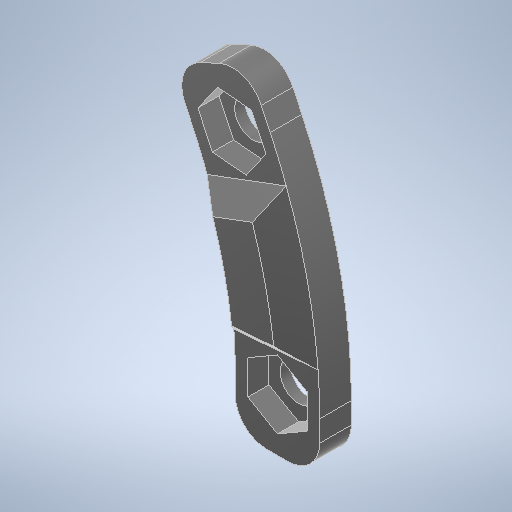
# Autodesk Inventor part: 3D_frame-connect-base2-2
Saved by Autodesk Inventor 2025 (Build 290162000, 162)
## iProperties
Created: 2024-07-30
Part Number: 3D_frame-connect-base2-2
Material: 一般
Document SubType Name: Modeling
Designer: 8326d
Density: 1 g/cm^3
Appearance: 滑らか - 黒
Author: 8326d
Autodesk Inventor part; units mm, degrees
ref_plane "YZ Plane" through (0, 0, 0) normal (1, 0, 0) x (0, 1, 0)
ref_plane "XZ Plane" through (0, 0, 0) normal (0, 1, 0) x (-1, 0, 0)
ref_plane "XY Plane" through (0, 0, 0) normal (0, 0, 1) x (1, 0, 0)
sketch "スケッチ1" plane through (0, 0, 0) normal (0, 0, 1) x (1, 0, 0)
  arc A0 (46, 0) -> (41.6902, 19.4404) centre (0, 0) ccw construction
  line L0 (0, 0) -> (46, 0) construction
  line L1 (0, 0) -> (46, 0) construction
  line L2 (0, 0) -> (41.6902, 19.4404) construction
  arc A1 (50, 0) -> (45.3154, 21.1309) centre (0, 0) ccw
  arc A2 (42, 0) -> (38.0649, 17.75) centre (0, 0) ccw
  line L3 (42, 0) -> (50, 0)
  line L4 (50, 0) -> (50, -5)
  line L5 (50, -5) -> (42, -5)
  line L6 (42, -5) -> (42, 0)
  line L7 (45.3154, 21.1309) -> (38.0649, 17.75)
  line L8 (38.0649, 17.75) -> (35.9518, 22.2815)
  line L9 (35.9518, 22.2815) -> (43.2023, 25.6625)
  line L10 (43.2023, 25.6625) -> (45.3154, 21.1309)
  dimension "d0" = 46
  dimension "d1" = 0
  dimension "d2" = 25
  dimension "d3" = 4
  dimension "d4" = 4
  dimension "d5" = 8
  dimension "d6" = 5
  dimension "d7" = 5
  constraints: 22 end point, 6 point on circle, 4 parallel, 4 point on line, 3 centre point, 3 coincident, 2 horizontal, 2 perpendicular, 1 collinear, 1 horizontal alignment
  measures "d0" radius of A0
  measures "d1" distance between parallel lines of L0 L1
  measures "d2" angle of L0 L2
  measures "d3" radial gap between concentric circles of A2 A0
  measures "d4" radial gap between concentric circles of A0 A1
  measures "d5" distance of L4.end L5.end
  measures "d6" distance of L3.end L4.end
  measures "d7" distance of L7.end L8.end
extrude "押し出し1" add sketch "スケッチ1" along normal blind 3
sketch "スケッチ2" plane through (0, 0, 3) normal (0, 0, 1) x (1, 0, 0)
  arc A0 (46, 0) -> (41.6902, 19.4404) centre (0, 0) ccw construction
  line L0 (0, 0) -> (46, 0) construction
  line L1 (0, 0) -> (46, 0) construction
  line L2 (0, 0) -> (41.6902, 19.4404) construction
  dimension "d10" = 46
  dimension "d11" = 0
  dimension "d12" = 25
  constraints: 6 end point, 3 coincident, 2 point on circle, 1 centre point, 1 collinear, 1 horizontal
  measures "d10" radius of A0
  measures "d11" distance between parallel lines of L0 L1
  measures "d12" angle of L0 L2
hole "穴1" at (41.6902, 19.4404, 3) at (46, 0, 3) direction (0, 0, -1) diameter 3.5 end through all
sketch "スケッチ3" plane through (0, 0, 3) normal (0, 0, 1) x (1, 0, 0)
  circle A0 centre (46, 0) radius 1.75 projected
  line L0 (46, 3.2332) -> (48.8, 1.6166)
  line L1 (48.8, 1.6166) -> (48.8, -1.6166)
  line L2 (48.8, -1.6166) -> (46, -3.2332)
  line L3 (46, -3.2332) -> (43.2, -1.6166)
  line L4 (43.2, -1.6166) -> (43.2, 1.6166)
  line L5 (43.2, 1.6166) -> (46, 3.2332)
  point P0 (0, 0)
  dimension "d20" = 5.6
  constraints: 12 end point, 1 coincident, 1 vertical alignment, 13 other
  measures "d20" distance between parallel lines of L1 L4
extrude "押し出し2" cut sketch "スケッチ3" against normal blind 2
pattern_circular "円形状パターン1" count 2 over 25 about axis through (0, 0, -10) along (0, 0, 1) of "押し出し2"
ref_plane "作業平面1" through (-22.5535, -5, 3) normal (-0.2164396, 0.976296, 0) x (0, 0, -1)
sketch "スケッチ4" plane through (-22.5535, -5, 3) normal (-0.2164396, 0.976296, 0) x (0, 0, -1)
  line L0 (3, -73.1011) -> (0, -73.1011) projected
  line L1 (0, -65.1011) -> (3, -65.1011) projected
  line L2 (0, -65.1011) -> (0, -64.1056) projected
  line L3 (0, -73.1011) -> (0, -65.1011)
  line L4 (0, -65.1011) -> (-2, -67.1011)
  line L5 (-2, -67.1011) -> (-2, -71.1011)
  line L6 (0, -71.9159) -> (0, -73.1011) projected
  line L7 (-2, -71.1011) -> (0, -73.1011)
  line L8 (4, -23.1011) -> (-3, -23.1011) projected
  point P0 (3, -23.1011)
  dimension "d26" = 45
  dimension "d27" = 45
  dimension "d28" = 2
  constraints: 8 end point, 1 parallel, 1 vertical
  measures "d26" angle of L3 L7
  measures "d27" angle of L3 L4
  measures "d28" distance between parallel lines of L3 L5
revolve "回転1" add sketch "スケッチ4" angle 16 mid plane about axis through (0, 0, -10) along (0, 0, 1)
chamfer "面取り1" distance 2 angle 45 2 edges at (43.0869, 16.1095, 5) (45.8582, 3.6091, 5)
fillet "フィレット1" radius 3 4 edges at (43.2023, 25.6625, 1.5) (35.9518, 22.2815, 1.5) (50, -5, 1.5) (42, -5, 1.5)
equation "\"d4\" = d3"
equation "\"d6\" = d7"
equation "\"d27\" = d26"
